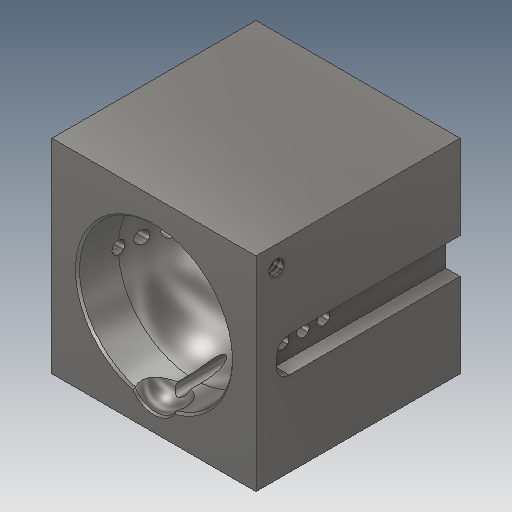
# Autodesk Inventor part: v2_nose_poke
Saved by Autodesk Inventor 2019 (Build 230136000, 136)
## iProperties
Created: 2017-09-27
Part Number: v2_nose_poke
Material: Stainless Steel
Document SubType Name: Modeling
Designer: richp
Density: 8 g/cm^3
Appearance: Semi-Polished
Mass: 99.3758 g
Surface Area: 51.5438 cm^2
Volume: 12.422 cm^3
Author: richp
Autodesk Inventor part; units mm, degrees
ref_plane "YZ Plane" through (0, 0, 0) normal (1, 0, 0) x (0, 1, 0)
ref_plane "XZ Plane" through (0, 0, 0) normal (0, 1, 0) x (-1, 0, 0)
sketch "Sketch1" plane through (0, 0, 0) normal (0, 0, 1) x (1, 0, 0)
  line L0 (-17.78, 0) -> (17.78, 0) projected
  line L1 (0, -5.08) -> (0, 30.48) projected
  line L2 (-12.7, 25.4) -> (12.7, 25.4)
  line L3 (12.7, 25.4) -> (12.7, 0)
  line L4 (12.7, 0) -> (-12.7, 0)
  line L5 (-12.7, 0) -> (-12.7, 25.4)
  point P0 (0, 0)
  dimension "d0" = 25.4
  dimension "d1" = 25.4
  constraints: 8 end point, 2 parallel, 1 horizontal, 1 perpendicular, 1 point on line, 1 other
  measures "d0" distance between parallel lines of L0 L2
  measures "d1" distance between parallel lines of L3 L5
extrude "Extrusion1" add sketch "Sketch1" against normal blind 25.4
sketch "Sketch2" plane through (0, 0, 0) normal (0, 0, 1) x (1, 0, 0)
  line L0 (12.7, 0) -> (12.7, 25.4) projected
  line L1 (12.7, 25.4) -> (-12.7, 25.4) projected
  line L2 (-12.7, 25.4) -> (-12.7, 0) projected
  line L3 (-12.7, 0) -> (12.7, 0) projected
  line L4 (0, -5.08) -> (0, 30.48) projected
  line L5 (-17.78, 0) -> (17.78, 0) projected
  circle A0 centre (0, 12.7) radius 9.525
  line L6 (0, 22.225) -> (0, 3.175)
  point P0 (0, 0)
  dimension "d4" = 19.05
  dimension "d5" = 12.7
  constraints: 2 end point, 2 point on circle, 2 point on line, 1 centre point, 1 midpoint
  measures "d4" diameter of A0
  measures "d5" distance from line of L3 A0.centre
extrude "Extrusion2" cut sketch "Sketch2" against normal blind 5.08 contours A0 L4 | L4 A0
sketch "Sketch4" plane through (0, 12.7, -5.08) normal (0, 0, 1) x (1, 0, 0)
  circle A0 centre (0, 0) radius 9.525 projected
  line L0 (0, 9.525) -> (0, -9.525)
  line L1 (12.7, -12.7) -> (12.7, 12.7) projected
  point P0 (0, -12.7)
  dimension "d10" = 12.7
  constraints: 2 end point, 2 point on circle, 1 vertical
  measures "d10" distance between parallel lines of L1 L0
revolve "Revolution2" cut sketch "Sketch4" angle 360 about axis through (0, 22.225, -5.08) along (0, -1, 0) picked at (3.3572, -2.7967) contours A0 L0
sketch "Sketch5" plane through (0, 0, -25.4) normal (0, 0, -1) x (-1, 0, 0)
  line L0 (-12.7, 0) -> (12.7, 0) projected
  line L1 (12.7, 0) -> (12.7, 25.4) projected
  point P0 (0, 0)
  point P1 (0, 3.175)
  dimension "d12" = 3.175
  dimension "d13" = 12.7
  measures "d12" distance from line of L0 point (0, 3.175)
  measures "d13" distance from line of L1 point (0, 3.175)
hole "Hole1" at (0, 3.175, -25.4) direction (0, 0, 1) diameter 1.6002 depth 25.4 tip angle 118
chamfer "Chamfer2" distance 0.254 angle 45 1 edges at (0, 22.225, 0)
ref_plane "Work Plane4" through (0, 0, 0) normal (1, 0, 0) x (0, 0, -1)
sketch "Sketch7" plane through (0, 0, 0) normal (1, 0, 0) x (0, 0, -1)
  line L0 (5.08, 3.2086) -> (0.254, 3.2086) construction
  line L1 (0, 0) -> (25.4, 0) construction
  line L2 (0, 0) -> (0, 25.4) construction
  circle A0 centre (1.27, 5.08) radius 3.175
  line L3 (1.27, 1.905) -> (1.27, 8.255)
  dimension "d41" = 5.08
  dimension "d42" = 1.27
  dimension "d43" = 6.35
  constraints: 2 end point, 2 point on circle, 1 centre point, 1 coincident, 1 midpoint, 1 vertical
  measures "d41" distance from line of L1 point (1.27, 5.08)
  measures "d42" distance from line of L2 point (1.27, 5.08)
  measures "d43" diameter of A0
revolve "Revolution3" cut sketch "Sketch7" angle 360 about axis through (0, 1.905, -1.27) along (0, 1, 0) picked at (2.0974, 5.7399) contours A0 L3
chamfer "Chamfer3" distance 0.254 angle 45 1 edges at (0, 2.1701, 0)
sketch "Sketch8" plane through (0, 0, -25.4) normal (0, 0, -1) x (-1, 0, 0)
  line L0 (12.7, 25.4) -> (-12.7, 25.4) projected
  line L1 (12.7, 0) -> (12.7, 25.4) projected
  point P0 (0, 0)
  point P1 (0, 15.875)
  dimension "d48" = 9.525
  dimension "d49" = 12.7
  measures "d48" distance from line of L0 point (0, 15.875)
  measures "d49" distance from line of L1 point (0, 15.875)
hole "Hole3" at (0, 15.875, -25.4) direction (0, 0, 1) diameter 1.6002 depth 25.4 tip angle 118
sketch "Sketch9" plane through (12.7, 0, 0) normal (1, 0, 0) x (0, 0, -1)
  line L0 (25.4, 0) -> (25.4, 25.4) construction
  line L1 (25.4, 12.7) -> (0, 12.7) construction
  line L2 (0, 0) -> (0, 25.4) construction
  line L3 (0, 0) -> (25.4, 0) construction
  line L4 (25.4, 25.4) -> (25.4, 0) construction
  line L5 (0, 0) -> (0, 25.4) construction
  line L6 (0, 0) -> (25.4, 0) construction
  line L7 (25.4, 25.4) -> (25.4, 0) construction
  line L8 (0, 25.4) -> (25.4, 25.4) construction
  line L9 (4.1275, 14.8971) -> (25.4, 14.8971)
  line L10 (25.4, 14.8971) -> (25.4, 10.5029)
  line L11 (25.4, 10.5029) -> (4.1275, 10.5029)
  line L12 (2.54, 12.0904) -> (2.54, 13.3096)
  arc A0 (2.54, 12.0904) -> (4.1275, 10.5029) centre (4.1275, 12.0904) ccw
  arc A1 (4.1275, 14.8971) -> (2.54, 13.3096) centre (4.1275, 13.3096) ccw
  point P0 (2.54, 14.8971)
  point P1 (2.54, 10.5029)
  dimension "d57" = 4.3942
  dimension "d58" = 0
  dimension "d59" = 2.54
  dimension "d62" = 1.5875
  constraints: 10 end point, 4 point on circle, 4 point on line, 4 tangent, 2 centre point, 2 horizontal, 2 midpoint, 2 parallel, 1 equal radius, 1 perpendicular, 1 other
  measures "d57" distance between parallel lines of L11 L9
  measures "d58" distance between parallel lines of L0 L10
  measures "d59" distance between parallel lines of L2 L12
  measures "d62" radius of A0
extrude "Extrusion3" cut sketch "Sketch9" against normal blind 1.778
sketch "Sketch10" plane through (-12.7, 0, 0) normal (-1, 0, 0) x (0, 0, 1)
  line L0 (-4.1275, 14.8971) -> (-25.4, 14.8971) projected
  arc A0 (-2.54, 13.3096) -> (-4.1275, 14.8971) centre (-4.1275, 13.3096) ccw projected
  line L1 (-2.54, 12.0904) -> (-2.54, 13.3096) projected
  arc A1 (-4.1275, 10.5029) -> (-2.54, 12.0904) centre (-4.1275, 12.0904) ccw projected
  line L2 (-25.4, 10.5029) -> (-4.1275, 10.5029) projected
  line L3 (-25.4, 14.8971) -> (-25.4, 10.5029) projected
  point P0 (0, 0)
extrude "Extrusion4" cut sketch "Sketch10" against normal blind 1.778
sketch "Sketch11" plane through (12.7, 0, 0) normal (1, 0, 0) x (0, 0, -1)
  line L0 (0, 25.4) -> (25.4, 25.4) projected
  line L1 (0, 0) -> (0, 25.4) projected
  line L2 (0, 0) -> (25.4, 0) projected
  point P0 (5.08, 12.7)
  point P1 (7.62, 12.7)
  point P2 (10.16, 12.7)
  dimension "d65" = 12.7
  dimension "d66" = 5.08
  dimension "d67" = 7.62
  dimension "d68" = 10.16
  dimension "d69" = 12.7
  constraints: 1 horizontal alignment
  measures "d65" distance from line of L0 point (5.08, 12.7)
  measures "d66" distance from line of L1 point (5.08, 12.7)
  measures "d67" distance from line of L1 point (7.62, 12.7)
  measures "d68" distance from line of L1 point (10.16, 12.7)
  measures "d69" distance from line of L2 point (10.16, 12.7)
hole "Hole4" at (12.7, 12.7, -5.08) at (12.7, 12.7, -7.62) at (12.7, 12.7, -10.16) direction (-1, 0, 0) diameter 1.6002 depth 25.4 tip angle 118
sketch "Sketch12" plane through (12.7, 0, 0) normal (1, 0, 0) x (0, 0, -1)
  line L0 (0, 25.4) -> (25.4, 25.4) projected
  line L1 (0, 0) -> (0, 25.4) projected
  point P0 (2.54, 22.86)
  dimension "d77" = 2.54
  dimension "d78" = 2.54
  measures "d77" distance from line of L0 point (2.54, 22.86)
  measures "d78" distance from line of L1 point (2.54, 22.86)
hole "Hole5" at (12.7, 22.86, -2.54) direction (-1, 0, 0) diameter 1.9304 depth 7.62 tip angle 118
sketch "Sketch13" plane through (-12.7, 0, 0) normal (-1, 0, 0) x (0, 0, 1)
  point P0 (0, 0)
  point P1 (-2.54, 22.86)
hole "Hole6" at (-12.7, 22.86, -2.54) direction (1, 0, 0) diameter 1.9304 depth 7.6708 tip angle 118
sketch "Sketch14" plane through (0, 0, -25.4) normal (0, 0, -1) x (-1, 0, 0)
  line L0 (0, -5.08) -> (0, 30.48) projected
  line L1 (10.16, 1.27) -> (-10.16, 1.27) construction
  line L2 (-10.16, 1.27) -> (-10.16, 19.05) construction
  line L3 (-10.16, 19.05) -> (10.16, 19.05) construction
  line L4 (10.16, 19.05) -> (10.16, 1.27) construction
  line L5 (10.16, 1.27) -> (-10.16, 19.05) construction
  line L6 (-10.16, 1.27) -> (10.16, 19.05) construction
  line L7 (-12.7, 0) -> (12.7, 0) construction
  point P0 (0, 0)
  point P1 (-7.62, 16.51)
  point P2 (7.62, 16.51)
  point P3 (0, 10.16)
  point P4 (0, 9.525)
  point P5 (0, 12.954)
  dimension "d93" = 15.24
  dimension "d94" = 17.78
  dimension "d95" = 20.32
  dimension "d96" = 10.16
  dimension "d97" = 2.54
  dimension "d98" = 8.255
  dimension "d113" = 11.684
  constraints: 12 end point, 3 point on line, 2 midpoint, 2 parallel, 1 horizontal, 1 perpendicular, 1 symmetric about line
  measures "d93" distance of point (7.62, 16.51) point (-7.62, 16.51)
  measures "d94" distance between parallel lines of L1 L3
  measures "d95" distance between parallel lines of L4 L2
  measures "d96" distance from line of L7 point (0, 10.16)
  measures "d97" distance from line of L3 point (7.62, 16.51)
  measures "d98" distance from line of L1 point (0, 9.525)
  measures "d113" distance from line of L1 point (0, 12.954)
hole "Hole7" at (0, 9.525, -25.4) direction (0, 0, 1) diameter 1.27 end through all
sketch "Sketch15" plane through (0, 0, -25.4) normal (0, 0, -1) x (-1, 0, 0)
  point P0 (0, 0)
  point P1 (-7.62, 16.51)
  point P2 (7.62, 16.51)
hole "Hole8" at (7.62, 16.51, -25.4) at (-7.62, 16.51, -25.4) direction (0, 0, 1) diameter 2.159 depth 8.8646 tip angle 118
sketch "Sketch16" plane through (0, 0, -25.4) normal (0, 0, -1) x (-1, 0, 0)
  point P0 (0, 0)
  point P1 (0, 12.954)
hole "Hole9" at (0, 12.954, -25.4) direction (0, 0, 1) diameter 3.81 depth 25.4 tip angle 118
body "Solid1"
